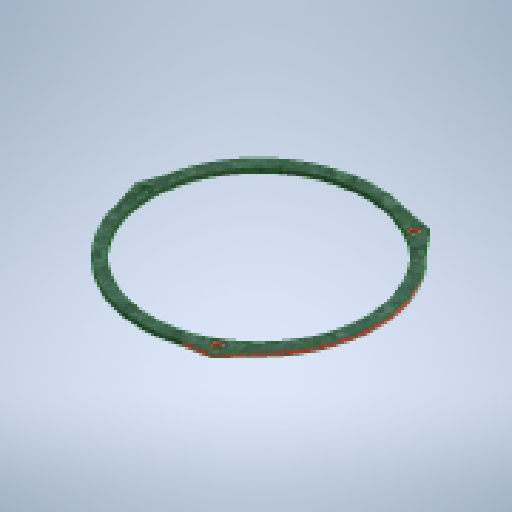
# Autodesk Inventor part: top
Saved by Autodesk Inventor 2023 (Build 270158000, 158)
## iProperties
Created: 2023-11-12
Part Number: top
Material: Ogólny
Document SubType Name: Modeling
Designer: janek
Density: 1 g/cm^3
Appearance: Domyślna
Author: janek
## iProperties of the stored document top_Drukowanie 3D.ipt
Created: 2023-11-13
Part Number: top_Drukowanie 3D
Material: Ogólny
Document SubType Name: Modeling
Designer: janek
Density: 1 g/cm^3
Appearance: Domyślna
Author: janek
Autodesk Inventor part; units mm, degrees
ref_plane "YZ Plane" through (0, 0, 0) normal (1, 0, 0) x (0, 1, 0)
ref_plane "XZ Plane" through (0, 0, 0) normal (0, 1, 0) x (-1, 0, 0)
ref_plane "XY Plane" through (0, 0, 0) normal (0, 0, 1) x (1, 0, 0)
sketch "Szkic1" plane through (0, 0, 0) normal (0, 1, 0) x (-1, 0, 0)
  circle A0 centre (0, 0) radius 145
  circle A1 centre (0, 0) radius 160
  dimension "d0" = 290
  dimension "d1" = 320
  constraints: 2 centre point, 2 coincident
  measures "d0" diameter of A0
  measures "d1" diameter of A1
extrude "Wyciągnięcie proste1" add sketch "Szkic1" along normal blind 6
sketch "Szkic2" plane through (0, 6, 0) normal (0, 1, 0) x (1, 0, 0)
  line L0 (-153.5, 0) -> (76.75, 132.9349)
  line L1 (76.75, 132.9349) -> (76.75, -132.9349)
  line L2 (76.75, -132.9349) -> (-153.5, 0)
  circle A0 centre (0, 0) radius 145 projected
  circle A1 centre (76.75, 132.9349) radius 4.25
  circle A2 centre (76.75, -132.9349) radius 4.25
  circle A3 centre (-153.5, 0) radius 4.25
  circle A4 centre (0, 0) radius 160 projected
  line L3 (-157.6376, -27.3932) -> (-167.6079, 0)
  line L4 (-167.6079, 0) -> (-157.6376, 27.3932)
  arc A5 (-157.6376, 27.3932) -> (-157.6376, -27.3932) centre (0, 0) ccw
  dimension "d4" = 60
  dimension "d5" = 153.5
  dimension "d6" = 153.5
  dimension "d7" = 153.5
  dimension "d8" = 60
  dimension "d9" = 8.5
  dimension "d10" = 8.5
  dimension "d11" = 8.5
  dimension "d14" = 140
  constraints: 10 end point, 4 centre point, 4 point on circle, 3 coincident, 1 concentric, 1 equal length, 1 vertical
  measures "d4" angle of L0 L2
  measures "d5" distance of A0.centre L0.start
  measures "d6" distance of L0.end point (0, 0)
  measures "d7" distance of point (0, 0) L1.end
  measures "d8" angle of L2 L1
  measures "d9" diameter of A1
  measures "d10" diameter of A2
  measures "d11" diameter of A3
  measures "d14" angle of L4 L3
extrude "Wyciągnięcie proste2" cut sketch "Szkic2" against normal blind 6 contours L2 A3 L0 | L0 A3 L2 | A1 L1 L0 | L0 L1 A1 | A2 L1 L2 | L2 L1 A2
extrude "Wyciągnięcie proste3" add sketch "Szkic2" against normal blind 6 contours A4 L3 L4
sketch "Szkic3" plane through (0, 6, 0) normal (0, 1, 0) x (1, 0, 0)
  arc A0 (-157.6376, -27.3932) -> (-157.6376, 27.3932) centre (0, 0) ccw projected
  line L0 (49.4646, 152.1619) -> (84.304, 146.0188)
  line L1 (84.304, 146.0188) -> (107.0438, 118.9185)
  circle A1 centre (76.75, 132.9349) radius 4.25 projected
  line L2 (49.4646, -152.1619) -> (84.304, -146.0188)
  line L3 (84.304, -146.0188) -> (107.0438, -118.9185)
  circle A2 centre (76.75, -132.9349) radius 4.25 projected
  line L4 (0, 0) -> (76.75, 132.9349)
  line L5 (84.304, 146.0188) -> (76.75, 132.9349)
  line L6 (76.75, -132.9349) -> (0, 0)
  line L7 (84.304, -146.0188) -> (76.75, -132.9349)
  dimension "d17" = 140
  dimension "d19" = 140
  dimension "d20" = 15.108
  dimension "d25" = 168.608
  constraints: 16 end point, 4 point on circle, 2 collinear, 2 equal length
  measures "d17" angle of L0 L1
  measures "d19" angle of L3 L2
  measures "d20" distance of L6.start L2.end
  measures "d25" distance of L0.end point (0, 0)
extrude "Wyciągnięcie proste4" add sketch "Szkic3" against normal blind 6 contours L3 L7 A0 | A0 L5 L1 | L7 L2 A0 | A0 L0 L5
fillet "Zaokrąglenie1" radius 3 3 edges at (72.5, 6, -132.9349) (72.5, 6, 132.9349) (-157.75, 6, 0) inverted yes
sketch "Szkic4" plane through (0, 0, 0) normal (0, -1, 0) x (1, 0, 0)
  line L0 (152.5, 0) -> (-76.2173, 132.05)
  line L1 (-76.2173, 132.05) -> (-76.2173, -132.05)
  line L2 (-76.2173, -132.05) -> (152.5, 0)
  arc A0 (107.0438, -118.9185) -> (107.0438, 118.9185) centre (0, 0) ccw projected
  arc A1 (-157.6376, -27.3932) -> (49.4646, -152.1619) centre (0, 0) ccw projected
  line L3 (160, 0) -> (0, 0)
  line L4 (-76.2173, 132.05) -> (38.1413, -66.025)
  line L5 (-76.2173, -132.05) -> (38.1413, 66.025)
  line L6 (152.5, 0) -> (-76.2173, 0)
  circle A2 centre (152.5, 0) radius 4
  circle A3 centre (-76.2173, -132.05) radius 4
  circle A4 centre (-76.2173, 132.05) radius 4
  line L7 (107.8338, 107.8338) -> (-107.8338, 107.8338)
  line L8 (-107.8338, 107.8338) -> (-107.8338, -107.8338)
  line L9 (-107.8338, -107.8338) -> (107.8338, -107.8338)
  line L10 (107.8338, -107.8338) -> (107.8338, 107.8338)
  line L11 (107.8338, 107.8338) -> (-107.8338, -107.8338) construction
  line L12 (-107.8338, 107.8338) -> (107.8338, -107.8338) construction
  circle A5 centre (107.8338, 107.8338) radius 4
  circle A6 centre (107.8338, -107.8338) radius 4
  circle A7 centre (-107.8338, 107.8338) radius 4
  circle A8 centre (-107.8338, -107.8338) radius 4
  dimension "d26" = 7.5
  dimension "d28" = 60
  dimension "d29" = 60
  dimension "d31" = 264.1
  dimension "d32" = 8
  dimension "d33" = 8
  dimension "d34" = 8
  dimension "d35" = 305
  dimension "d37" = 8
  dimension "d38" = 8
  dimension "d39" = 8
  dimension "d40" = 8
  constraints: 26 end point, 7 centre point, 7 coincident, 5 midpoint, 2 horizontal, 2 parallel, 2 perpendicular, 1 point on circle, 1 point on line, 1 vertical
  measures "d26" distance of L3.start L0.start
  measures "d28" angle of L2 L0
  measures "d29" angle of L0 L1
  measures "d31" distance of L0.end L1.end
  measures "d32" diameter of A2
  measures "d33" diameter of A3
  measures "d34" diameter of A4
  measures "d35" distance of L7.start L8.end
  measures "d37" diameter of A5
  measures "d38" diameter of A6
  measures "d39" diameter of A7
  measures "d40" diameter of A8
extrude "Wyciągnięcie proste6" cut sketch "Szkic4" against normal blind 2.5 contours L3 A2 L0 | L3 A2 L2 | L0 A2 L3 | L2 A2 L3 | A5 L7 L10 | L10 L7 A5 | A6 L9 L10 | L10 L9 A6 | A4 L4 L0 | L0 L1 A4 | A3 L1 L2 | L2 L5 A3 | A4 L1 L4 | L5 L1 A3 | A7 L8 L7 | L7 L8 A7 | A8 L8 L9 | L9 L8 A8
